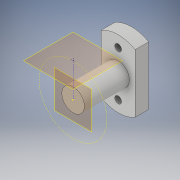
# Autodesk Inventor part: spannring_achse_lager
Saved by Autodesk Inventor 2017 (Build 210142000, 142)
## iProperties
Part Number: spannring_achse_lager
Material: Generisch
Document SubType Name: Modeling
Designer: Fabio
Density: 1 g/cm^3
Appearance: Vorgabe
Author: Fabio
Autodesk Inventor part; units mm, degrees
ref_plane "YZ Plane" through (0, 0, 0) normal (1, 0, 0) x (0, 1, 0)
ref_plane "XZ Plane" through (0, 0, 0) normal (0, 1, 0) x (-1, 0, 0)
ref_plane "XY Plane" through (0, 0, 0) normal (0, 0, 1) x (1, 0, 0)
sketch "Skizze1" plane through (0, 0, 0) normal (0, 1, 0) x (-1, 0, 0)
  circle A0 centre (0, 0) radius 15
  dimension "d0" = 30
  constraints: 1 centre point, 1 coincident
  measures "d0" diameter of A0
extrude "Extrusion1" add sketch "Skizze1" along normal blind 26
ref_plane "Arbeitsebene1" through (0, 26, 0) normal (0, 1, 0) x (1, 0, 0)
sketch "Skizze2" plane through (0, 26, 0) normal (0, 1, 0) x (1, 0, 0)
  circle A0 centre (0, 0) radius 15 projected
  circle A1 centre (0, 0) radius 15 construction
  circle A2 centre (0, 0) radius 15 construction
  line L0 (0, 0) -> (0, 10) construction
  line L1 (0, 0) -> (0, -10) construction
  dimension "d4" = 10
  dimension "d5" = 10
  constraints: 4 end point, 2 vertical
  measures "d4" distance of point (0, 0) L1.end
  measures "d5" distance of L0.end point (0, 0)
hole "Bohrung1" at (0, 26, 10) at (0, 26, -10) direction (0, -1, 0) diameter 3 end through all
thread "Gewinde1" size "M3x0.5" class "6H" standard "ANSI Metric M Profile" full length
thread "Gewinde2" size "M3x0.5" class "6H" standard "ANSI Metric M Profile" full length
ref_plane "Arbeitsebene2" through (0, 0, 0) normal (0, -1, 0) x (1, 0, 0)
sketch "Skizze4" plane through (0, 0, 0) normal (0, -1, 0) x (1, 0, 0)
  point P0 (0, 0)
sketch "Skizze5" plane through (0, 0, 0) normal (0, -1, 0) x (1, 0, 0)
  line L0 (0, 0) -> (0, 15) construction
  circle A0 centre (0, 0) radius 15 construction
  constraints: 2 end point, 1 coincident, 1 vertical, 1 vertical alignment, 1 other
ref_plane "Arbeitsebene3" through (0, 0, 15) normal (0, 0, 1) x (1, 0, 0)
sketch "Skizze7" plane through (0, 0, 0) normal (0, -1, 0) x (1, 0, 0)
  circle A0 centre (0, 0) radius 5
  circle A1 centre (0, 0) radius 20
  dimension "d38" = 10
  dimension "d39" = 40
  constraints: 2 centre point, 2 coincident
  measures "d38" diameter of A0
  measures "d39" diameter of A1
extrude "Extrusion2" cut sketch "Skizze7" against normal blind 20
sketch "Skizze8" plane through (0, 20, 0) normal (0, -1, 0) x (1, 0, 0)
  line L0 (-7.5, -17.5) -> (7.5, -17.5)
  line L1 (7.5, -17.5) -> (7.5, 17.5)
  line L2 (7.5, 17.5) -> (-7.5, 17.5)
  line L3 (-7.5, 17.5) -> (-7.5, -17.5)
  line L4 (-7.5, -17.5) -> (7.5, 17.5) construction
  line L5 (7.5, -17.5) -> (-7.5, 17.5) construction
  point P0 (0, 0)
  dimension "d42" = 15
  dimension "d43" = 35
  constraints: 12 end point, 2 midpoint, 2 parallel, 1 horizontal, 1 perpendicular
  measures "d42" distance of L2.end L1.end
  measures "d43" distance of L1.end L0.end
extrude "Extrusion3" cut sketch "Skizze8" along normal through all both and the other way through all keep common part
